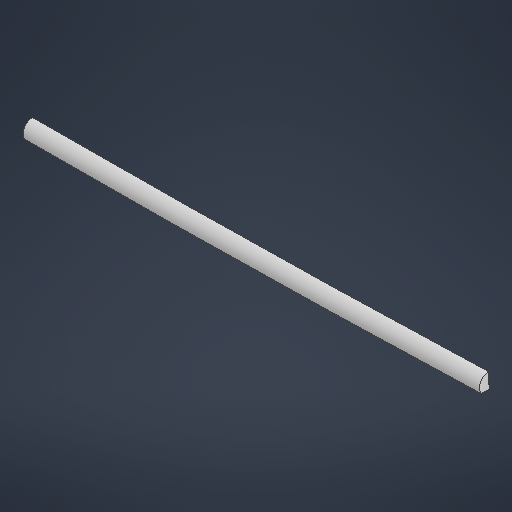
# Autodesk Inventor part: Peça1
Saved by Autodesk Inventor 2027 (Build 310192000, 192)
## iProperties
Created: 2025-11-26
Part Number: Peça1
Material: Genérico
Document SubType Name: Modeling
Designer: Lucas David
Density: 1 g/cm^3
Appearance: Padrão
Author: Lucas David
Autodesk Inventor part; units mm, degrees
ref_plane "YZ Plane" through (0, 0, 0) normal (1, 0, 0) x (0, 1, 0)
ref_plane "XZ Plane" through (0, 0, 0) normal (0, 1, 0) x (-1, 0, 0)
ref_plane "XY Plane" through (0, 0, 0) normal (0, 0, 1) x (1, 0, 0)
sketch "Esboço2" plane through (0, 0, 0) normal (1, 0, 0) x (0, 1, 0)
  circle A0 centre (0, 0) radius 0.0041
  arc A1 (-0.035, -0.0518) -> (-0.035, 0.0518) centre (0, 0) ccw
  line L0 (-0.035, 0.0518) -> (-0.035, -0.0518)
  dimension "d15" = 0.125
  dimension "d16" = 0.0082
  dimension "d17" = 0.035
  constraints: 2 centre point, 2 end point, 2 point on circle, 1 coincident, 1 vertical
  measures "d15" diameter of A1
  measures "d16" diameter of A0
  measures "d17" distance from line of L0 A0.centre
sketch "Esboço1" plane through (0, 0, 0) normal (0, 0, 1) x (1, 0, 0)
  line L0 (0, 0) -> (3, 0.0524) construction
  line L1 (0, 0) -> (3, 0) construction
  arc A0 (0, 0) -> (3, 0.0524) centre (0, 85.9611) ccw
  dimension "d0" = 1
  dimension "d1" = 3
  constraints: 4 end point, 2 point on circle, 1 centre point, 1 horizontal, 1 tangent, 1 vertical alignment
  measures "d0" angle of L1 L0
  measures "d1" distance of L0.start L1.end
sweep "Varredura4" add profiles "Esboço2" path "Esboço1"
sketch "Esboço4" plane through (0, 0, 0) normal (0, 0, 1) x (1, 0, 0)
  line L0 (3.0802, 0.5654) -> (-0.2032, 0.5654)
  line L1 (-0.2032, 0.5654) -> (-0.2032, -0.5119)
  line L2 (-0.2032, -0.5119) -> (3.0802, -0.5119)
  line L3 (3.0802, -0.5119) -> (3.0802, 0.5654)
  point P0 (0, 0)
  constraints: 8 end point, 2 parallel, 1 horizontal, 1 perpendicular
extrude "Extrusão2" cut sketch "Esboço4" against normal blind 10
